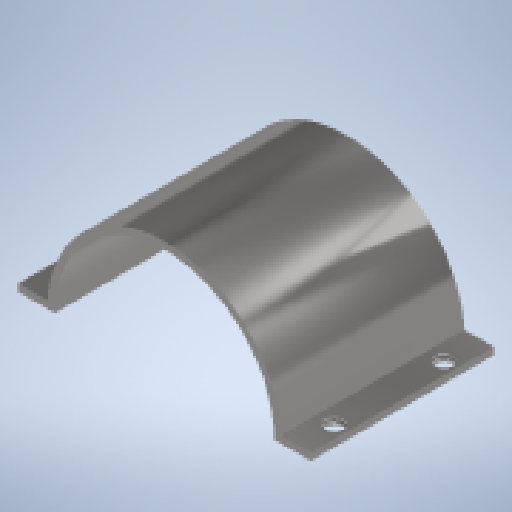
# Autodesk Inventor part: Peça2
Saved by Autodesk Inventor 2026 (Build 300175000, 175)
## iProperties
Created: 2025-11-26
Part Number: Peça2
Material: Genérico
Document SubType Name: Sheet Metal
Designer: rafae
Density: 1 g/cm^3
Sheet Metal Rule: Default_mm
Appearance: Aço - Polido
Author: rafae
Autodesk Inventor part; units mm, degrees
ref_plane "YZ Plane" through (0, 0, 0) normal (1, 0, 0) x (0, 1, 0)
ref_plane "XZ Plane" through (0, 0, 0) normal (0, 1, 0) x (-1, 0, 0)
ref_plane "XY Plane" through (0, 0, 0) normal (0, 0, 1) x (1, 0, 0)
sketch "Esboço1" plane through (0, 0, 0) normal (0, 0, 1) x (1, 0, 0)
  line L0 (0, 0) -> (-2, 0)
  arc A0 (-2, 0) -> (-14, 0) centre (-8, 0) ccw
  line L1 (-14, 0) -> (-16, 0)
  line L2 (-16, 0.4) -> (-14.3875, 0.4)
  arc A1 (-1.6125, 0.4) -> (-14.3875, 0.4) centre (-8, 0) ccw
  line L3 (-1.6125, 0.4) -> (0, 0.4)
  line L4 (0, 0.4) -> (0, 0)
  line L5 (-16, 0.4) -> (-16, 0)
  dimension "d2" = 2
  dimension "d3" = 12
  dimension "d4" = 6
  dimension "d5" = 2
  dimension "d6" = 6.4
  constraints: 12 end point, 4 point on circle, 2 centre point, 2 horizontal, 1 perpendicular, 1 point on line, 1 vertical, 2 other
  measures "d2" distance of L0.start L0.end
  measures "d3" distance of L0.end L1.start
  measures "d4" radius of A0
  measures "d5" distance of L1.start L1.end
  measures "d6" radius of A1
extrude "Extrusão1" add sketch "Esboço1" along normal mid plane 10
sketch "Esboço4" plane through (-1.6125, 0.4, 5) normal (0, 1, 0) x (1, 0, 0)
  line L0 (1.6125, 10) -> (1.6125, 0) projected
  line L1 (1.6125, 0) -> (0, 0) projected
  line L2 (0, 10) -> (1.6125, 10) projected
  point P0 (1.6125, 5)
  point P1 (0.9125, 2)
  point P2 (0.9125, 8)
  point P3 (0.8063, 0)
  dimension "d13" = 0.7
  dimension "d14" = 0.7
  dimension "d15" = 2
  dimension "d16" = 2
  constraints: 1 midpoint
  measures "d13" distance from line of L0 point (0.913, 2)
  measures "d14" distance from line of L0 point (0.913, 8)
  measures "d15" vertical distance of point (0.806, 0) point (0.913, 2)
  measures "d16" distance from line of L2 point (0.913, 8)
hole "Furo1" at (-0.7, 0.4, 3) at (-0.7, 0.4, -3) direction (0, -1, 0) diameter 0.5 end through all counterbore diameter 1 counterbore depth 1
sketch "Esboço5" plane through (-16, 0.4, 5) normal (0, 1, 0) x (1, 0, 0)
  line L0 (0, 10) -> (0, 0) projected
  line L1 (0, 10) -> (1.6125, 10) projected
  line L2 (1.6125, 0) -> (0, 0) projected
  point P0 (16, 5)
  point P1 (0.7, 8)
  point P2 (0.7, 2)
  dimension "d24" = 0.7
  dimension "d25" = 2
  dimension "d26" = 2
  dimension "d27" = 0.7
  measures "d24" distance from line of L0 point (0.7, 8)
  measures "d25" distance from line of L1 point (0.7, 8)
  measures "d26" distance from line of L2 point (0.7, 2)
  measures "d27" distance from line of L0 point (0.7, 2)
hole "Furo2" at (-15.3, 0.4, -3) at (-15.3, 0.4, 3) direction (0, -1, 0) diameter 0.5 end through all counterbore diameter 1 counterbore depth 1
thread "Rosca1" size "M1x0.25" class "6H" standard "ANSI Metric M Profile" length 150
thread "Rosca2" size "M1x0.25" class "6H" standard "ANSI Metric M Profile" full length
thread "Rosca3" size "M1x0.25" class "6H" standard "ANSI Metric M Profile" full length
thread "Rosca4" size "M1x0.25" class "6H" standard "ANSI Metric M Profile" full length
thread "Rosca5" size "M1x0.25" class "6H" standard "ANSI Metric M Profile" full length
equation "\"Raio_vergadura\" = Espessura"
equation "\"Largura_alívio_de_vergadura\" = Espessura"
equation "\"Profundidade_alívio_de_vergadura\" = 0.5 * Espessura"
equation "\"Tamanho_alívio_de_dobra\" = 4 * Espessura"
equation "\"Remanescente_mínimo\" = 2 * Espessura"
equation "\"Raiodetransição\" = Raio_vergadura"
equation "\"Tamanho_de_raio_de_Jacobi\" = Raio_vergadura"
equation "\"TamanhoFolga\" = Espessura"
equation "\"Espessura\" = 0.5"
